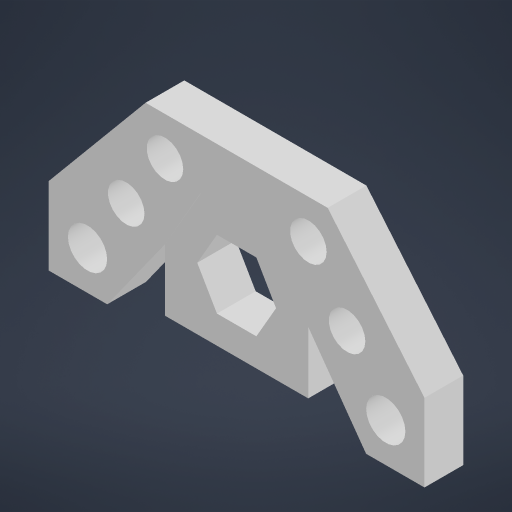
# Autodesk Inventor part: WireGuideBoltHols
Saved by Autodesk Inventor 2024.1 (Build 281209000, 209)
## iProperties
Created: 2023-08-17
Part Number: WireGuideBoltHols
Material: Generic
Document SubType Name: Modeling
Designer: Eleanor
Density: 1 g/cm^3
Appearance: Default
Author: Eleanor
Autodesk Inventor part; units mm, degrees
ref_plane "YZ Plane" through (0, 0, 0) normal (1, 0, 0) x (0, 1, 0)
ref_plane "XZ Plane" through (0, 0, 0) normal (0, 1, 0) x (-1, 0, 0)
ref_plane "XY Plane" through (0, 0, 0) normal (0, 0, 1) x (1, 0, 0)
sketch "Sketch1" plane through (0, 0, 0) normal (0, 0, 1) x (1, 0, 0)
  circle A0 centre (0, 0) radius 2.2479
  circle A1 centre (-1.3525, -2.3427) radius 0.4572
  circle A2 centre (1.3526, -2.3427) radius 0.4572
  circle A3 centre (2.7051, 0) radius 0.4572
  circle A4 centre (1.3525, 2.3427) radius 0.4572
  circle A5 centre (-1.3525, 2.3427) radius 0.4572
  circle A6 centre (-2.7051, 0) radius 0.4572
  line L0 (-1.6165, -2.7999) -> (-3.233, 0)
  line L1 (-3.233, 0) -> (-1.6165, 2.7999)
  line L2 (-1.6165, 2.7999) -> (1.6165, 2.7999)
  line L3 (1.6165, 2.7999) -> (3.233, 0)
  line L4 (3.233, 0) -> (1.6165, -2.7999)
  line L5 (1.6165, -2.7999) -> (-1.6165, -2.7999)
  line L6 (0, 0) -> (0, -5.0828)
  line L7 (-5.8691, 0) -> (-2.9345, 5.0828)
  line L8 (-2.9345, 5.0828) -> (2.9345, 5.0828)
  line L9 (2.9345, 5.0828) -> (5.8691, 0)
  line L10 (2.9345, -5.0828) -> (-2.9345, -5.0828)
  line L11 (-2.9345, -5.0828) -> (-5.8691, -5.0828)
  line L12 (-5.8691, -5.0828) -> (-5.8691, 0)
  line L13 (2.9345, -5.0828) -> (5.8691, -5.0828)
  line L14 (5.8691, -5.0828) -> (5.8691, 0)
  point P0 (0, -2.2479)
  dimension "d0" = 4.4958
  dimension "d4" = 360
  constraints: 30 end point, 6 centre point, 3 coincident, 2 perpendicular, 1 horizontal, 1 midpoint, 1 point on line, 1 vertical, 1 vertical alignment, 37 other
extrude "Extrusion1" add sketch "Sketch1" along normal blind 3.175
sketch "Sketch2" plane through (0, 0, 3.175) normal (0, 0, 1) x (1, 0, 0)
  line L0 (2.9345, 5.0828) -> (-2.9345, 5.0828) projected
  circle A0 centre (-9.0556, 1.3104) radius 1.5
  circle A1 centre (-5.8806, 6.0729) radius 1.5
  circle A2 centre (-12.2306, -3.4521) radius 1.6091
  line L1 (0, 0.0421) -> (0, 5.1689)
  circle A3 centre (9.0556, 1.3104) radius 1.5
  circle A4 centre (12.2306, -3.4521) radius 1.6091
  circle A5 centre (5.8806, 6.0729) radius 1.5
  line L2 (-5.8537, 0.0266) -> (-10.6162, -6.6427)
  line L3 (-10.6162, -6.6427) -> (-15.4056, -6.6427)
  line L4 (-15.4056, -6.6427) -> (-15.4056, -0.2771)
  line L5 (-15.4056, -0.2771) -> (-7.4681, 9.2479)
  line L6 (-7.4681, 9.2479) -> (0, 9.2479)
  line L7 (5.8537, 0.0266) -> (10.6162, -6.6427)
  line L8 (10.6162, -6.6427) -> (15.4056, -6.6427)
  line L9 (15.4056, -6.6427) -> (15.4056, -0.2771)
  line L10 (15.4056, -0.2771) -> (7.4681, 9.2479)
  line L11 (7.4681, 9.2479) -> (0, 9.2479)
  line L12 (5.8691, 0) -> (2.9345, 5.0828) projected
  line L13 (5.8537, 0.0266) -> (2.9345, 5.0828)
  line L14 (2.9345, 5.0828) -> (-2.9579, 5.0828)
  line L15 (5.8691, 0) -> (2.9345, 5.0828)
  line L16 (-2.9579, 5.0828) -> (-5.8537, 0.0266)
  dimension "d28" = 3
  dimension "d29" = 3
  dimension "d30" = 9.144
  constraints: 30 end point, 8 symmetric about line, 6 centre point, 1 collinear, 1 perpendicular, 1 point on line, 1 vertical, 3 other
  measures "d28" diameter of A0
  measures "d29" diameter of A1
  measures "d30" distance of A0.centre L1.start
ref_plane "Work Plane2" through (-2.9345, 5.0828, 0) normal (-0.8660254, -0.5, 0) x (0, 0, 1)
ref_plane "Work Plane3" through (0, 0, 1.5875) normal (0, 0, 1) x (1, 0, 0)
extrude "Extrusion4" add sketch "Sketch2" against normal blind 3.175
body "Solid1"
